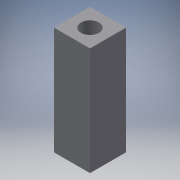
# Autodesk Inventor part: cilindro sierra
Saved by Autodesk Inventor 2018 (Build 220112000, 112)
## iProperties
Created: 2021-07-10
Part Number: cilindro sierra
Material: Genérico
Document SubType Name: Modeling
Designer: GABRIEL
Density: 1 g/cm^3
Appearance: Valor por defecto
Author: GABRIEL
Autodesk Inventor part; units mm, degrees
ref_plane "YZ Plane" through (0, 0, 0) normal (1, 0, 0) x (0, 1, 0)
ref_plane "XZ Plane" through (0, 0, 0) normal (0, 1, 0) x (-1, 0, 0)
ref_plane "XY Plane" through (0, 0, 0) normal (0, 0, 1) x (1, 0, 0)
sketch "Boceto1" plane through (0, 0, 0) normal (0, 0, 1) x (1, 0, 0)
  line L0 (0, 0) -> (40, 0)
  line L1 (40, 0) -> (40, -40)
  line L2 (40, -40) -> (0, -40)
  line L3 (0, -40) -> (0, 0)
  dimension "d0" = 40
  dimension "d1" = 40
  constraints: 8 end point, 2 parallel, 1 horizontal, 1 perpendicular
  measures "d0" distance of L1.end L2.end
  measures "d1" distance of L0.end L1.end
extrude "Extrusión1" add sketch "Boceto1" along normal blind 120
sketch "Boceto2" plane through (0, 0, 120) normal (0, 0, 1) x (1, 0, 0)
  circle A0 centre (20, -20) radius 10
  line L0 (0, 0) -> (0, -40) projected
  line L1 (40, 0) -> (0, 0) projected
  dimension "d4" = 20
  dimension "d5" = 20
  dimension "d6" = 20
  constraints: 1 centre point
  measures "d4" diameter of A0
  measures "d5" distance from line of L0 A0.centre
  measures "d6" distance from line of L1 A0.centre
extrude "Extrusión2" cut sketch "Boceto2" against normal blind 100
ref_plane "Plano de trabajo1" through (20, -40, 0) normal (-1, 0, 0) x (0, 0, 1)
sketch "Boceto5" plane through (20, -40, 0) normal (-1, 0, 0) x (0, 0, 1)
  line L0 (0, 0) -> (0, 40) projected
  line L1 (0, 30) -> (-15, 30)
  line L2 (-15, 30) -> (-15, 10)
  line L3 (-15, 10) -> (0, 10)
  line L4 (0, 10) -> (0, 30)
  line L5 (0, 40) -> (120, 40) projected
  circle A0 centre (-15, 20) radius 10
  dimension "d10" = 15
  dimension "d11" = 20
  dimension "d12" = 30
  constraints: 8 end point, 2 parallel, 1 horizontal, 1 midpoint, 1 perpendicular, 1 point on line, 1 vertical alignment, 2 other
  measures "d10" distance of L3.end L2.end
  measures "d11" distance of L2.end L1.end
  measures "d12" distance between parallel lines of L5 L3
extrude "Extrusión3" add sketch "Boceto5" along normal mid plane 12
hole "Agujero1" at (14, -19.1963, -18.9315) direction (1, 0, 0) diameter 8 end through all
